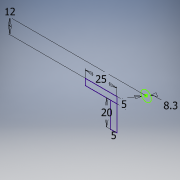
# Autodesk Inventor part: MA20 Top Connector
Saved by Autodesk Inventor 2019.4 (Build 234330000, 330)
## iProperties
Created: 2020-03-11
Part Number: MA20 Top Connector
Material: Generic
Document SubType Name: Modeling
Designer: Mark
Density: 1 g/cm^3
Appearance: Default
Author: Mark
Autodesk Inventor part; units mm, degrees
ref_plane "YZ Plane" through (0, 0, 0) normal (1, 0, 0) x (0, 1, 0)
ref_plane "XZ Plane" through (0, 0, 0) normal (0, 1, 0) x (-1, 0, 0)
ref_plane "XY Plane" through (0, 0, 0) normal (0, 0, 1) x (1, 0, 0)
sketch "Sketch1" plane through (0, 0, 0) normal (0, 0, 1) x (1, 0, 0)
  line L0 (0, 0) -> (25, 0)
  line L1 (25, 0) -> (25, 5)
  line L2 (25, 5) -> (0, 5)
  line L3 (0, 5) -> (0, 0)
  line L4 (25, 0) -> (20, 0)
  line L5 (20, 0) -> (20, -20)
  line L6 (20, -20) -> (25, -20)
  line L7 (25, -20) -> (25, 0)
  circle A0 centre (57.3, -14) radius 4.15
  circle A1 centre (57.3, -14) radius 10
  line L8 (25, 5) -> (59.8862, -4.3402)
  line L9 (25, -20) -> (56.047, -23.9212)
  dimension "d0" = 25
  dimension "d1" = 5
  dimension "d2" = 5
  dimension "d3" = 20
  dimension "d4" = 8.3
  dimension "d6" = 14
  dimension "d7" = 37.3
  dimension "d8" = 20
  constraints: 20 end point, 4 parallel, 2 centre point, 2 horizontal, 2 perpendicular, 2 point on circle, 2 tangent, 1 coincident
  measures "d0" distance of L2.end L1.end
  measures "d1" distance of L1.end L0.end
  measures "d2" distance of L6.end L5.end
  measures "d3" distance of L5.end L4.end
  measures "d4" diameter of A0
  measures "d6" distance from line of A0.centre L0
  measures "d7" distance from line of A0.centre L5
  measures "d8" diameter of A1
extrude "Extrusion1" add sketch "Sketch1" along normal blind 24 contours L3 L2 L1 L0 | L0 L7 L6 L5 | L1 L8 A1 L9 L7 | A1 | A0
sketch "Sketch2" plane through (0, 0, 24) normal (0, 0, 1) x (1, 0, 0)
  circle A0 centre (57.3, -14) radius 4.15
  arc A1 (56.047, -23.9212) -> (59.8862, -4.3402) centre (57.3, -14) ccw projected
  point P0 (0, 0)
  dimension "d11" = 8.3
  constraints: 1 centre point, 1 concentric
  measures "d11" diameter of A0
extrude "Extrusion2" cut sketch "Sketch2" against normal up to next
fillet "Fillet1" radius 5 2 edges at (25, -20, 12) (25, 5, 12)
sketch "Sketch3" plane through (59.8862, -4.3402, 24) normal (0.2586, 0.966, 0) x (0.966, -0.2586, 0)
  line L0 (10, 5.75) -> (-10, 5.75)
  line L1 (-10, 5.75) -> (-10, 18.25)
  line L2 (-10, 18.25) -> (10, 18.25)
  line L3 (10, 18.25) -> (10, 5.75)
  line L4 (0, 0) -> (-35.4572, 0) projected
  line L5 (0, 24) -> (0, 0) projected
  point P0 (-58.9713, 24)
  dimension "d15" = 20
  dimension "d16" = 12.5
  dimension "d17" = 5.75
  dimension "d18" = 10
  constraints: 8 end point, 2 parallel, 1 horizontal, 1 perpendicular
  measures "d15" distance of L1.end L2.end
  measures "d16" distance of L0.end L1.end
  measures "d17" distance between parallel lines of L4 L0
  measures "d18" distance between parallel lines of L5 L3
extrude "Extrusion3" cut sketch "Sketch3" against normal blind 24
sketch "Sketch4" plane through (0, 0, 24) normal (0, 0, 1) x (1, 0, 0)
  line L0 (24.3422, 5) -> (0, 5) projected
  line L1 (0, 5) -> (25, 5)
  line L2 (25, 5) -> (25, 0)
  line L3 (25, 0) -> (0, 0)
  line L4 (0, 0) -> (0, 5)
  line L5 (25, 0) -> (20, 0)
  line L6 (20, 0) -> (20, -20)
  line L7 (20, -20) -> (25, -20)
  line L8 (25, -20) -> (25, 0)
  dimension "d21" = 25
  dimension "d22" = 5
  dimension "d23" = 5
  dimension "d24" = 20
  constraints: 16 end point, 4 parallel, 2 horizontal, 2 perpendicular
  measures "d21" distance of L2.end L3.end
  measures "d22" distance of L1.end L2.end
  measures "d23" distance of L7.end L6.end
  measures "d24" distance of L6.end L5.end
extrude "Extrusion4" add sketch "Sketch4" along normal blind 30 and the other way blind 54
sketch "Sketch5" plane through (25, -20, 24) normal (1, 0, 0) x (0, 0, -1)
  circle A0 centre (-15, 10) radius 2.75
  circle A1 centre (39, 10) radius 2.75
  line L0 (-30, 0) -> (0, 0) projected
  line L1 (24, 0) -> (54, 0) projected
  line L2 (54, 25) -> (54, 0) projected
  line L3 (-30, 0) -> (-30, 25) projected
  point P0 (24, 20)
  dimension "d29" = 5.5
  dimension "d30" = 5.5
  dimension "d31" = 10
  dimension "d32" = 10
  dimension "d33" = 15
  dimension "d34" = 15
  constraints: 2 centre point
  measures "d29" diameter of A0
  measures "d30" diameter of A1
  measures "d31" distance from line of L0 A0.centre
  measures "d32" distance from line of L1 A1.centre
  measures "d33" distance from line of L2 A1.centre
  measures "d34" distance from line of L3 A0.centre
extrude "Extrusion5" cut sketch "Sketch5" against normal blind 30
sketch "Sketch6" plane through (0, 5, 54) normal (0, 1, 0) x (1, 0, 0)
  circle A0 centre (10, 15) radius 2.75
  circle A1 centre (10, 69) radius 2.75
  line L0 (25, 0) -> (25, 84) projected
  line L1 (0, 84) -> (25, 84) projected
  line L2 (0, 84) -> (0, 0) projected
  line L3 (25, 0) -> (0, 0) projected
  point P0 (0, 54)
  dimension "d37" = 5.5
  dimension "d38" = 5.5
  dimension "d39" = 15
  dimension "d40" = 15
  dimension "d41" = 10
  dimension "d42" = 15
  constraints: 2 centre point
  measures "d37" diameter of A0
  measures "d38" diameter of A1
  measures "d39" distance from line of L0 A1.centre
  measures "d40" distance from line of L1 A1.centre
  measures "d41" distance from line of L2 A0.centre
  measures "d42" distance from line of L3 A0.centre
extrude "Extrusion6" cut sketch "Sketch6" against normal blind 30 contours A0 | A1
equation "\"d12\" = d11"
body "Solid1"
